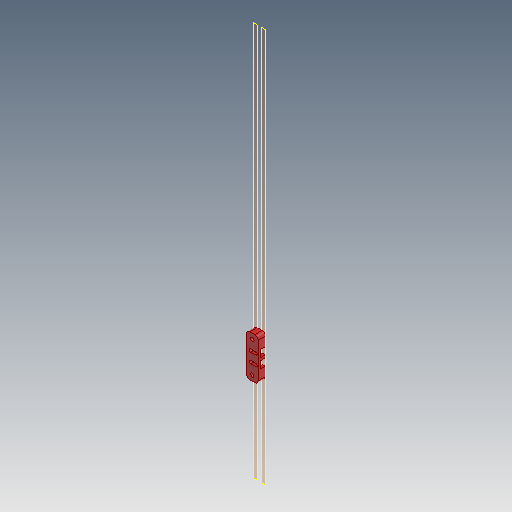
# Autodesk Inventor part: Limit swtich mount bottom
Saved by Autodesk Inventor 2020 (Build 240168000, 168)
## iProperties
Created: 2019-11-21
Part Number: Limit swtich mount bottom
Material: Generic
Document SubType Name: Modeling
Designer: ball
Density: 1 g/cm^3
Appearance: Default
Author: ball
Autodesk Inventor part; units mm, degrees
ref_plane "YZ Plane" through (0, 0, 0) normal (1, 0, 0) x (0, 1, 0)
ref_plane "XZ Plane" through (0, 0, 0) normal (0, 1, 0) x (-1, 0, 0)
ref_plane "Work Plane1" through (0, 0, 0) normal (0, 0, 1) x (1, 0, 0)
ref_plane "Work Plane2" through (0, 0, 0) normal (0, 0, 1) x (1, 0, 0)
sketch "Sketch2" plane through (0, 0, 0) normal (0, 0, 1) x (1, 0, 0)
  line L0 (1.9142, -654.4) -> (1.9142, -1000) construction
  line L1 (13.0858, -1000) -> (13.0858, -654.4) construction
  line L2 (10.8204, -900) -> (1.905, -900) construction
  line L3 (1.1684, -919.8882) -> (10.8204, -919.8882) construction
  circle A0 centre (8.3884, -914.7066) radius 1.1938 construction
  circle A1 centre (8.3884, -905.1816) radius 1.1938 construction
  line L4 (1.9142, -930.0482) -> (13.0858, -930.0482)
  line L5 (13.0858, -930.0482) -> (13.0858, -889.84)
  line L6 (13.0858, -889.84) -> (1.9142, -889.84)
  line L7 (1.9142, -889.84) -> (1.9142, -930.0482)
  circle A2 centre (7.5, -924.8932) radius 1.7
  circle A3 centre (7.5, -894.995) radius 1.7
  circle A4 centre (5.8484, -914.7066) radius 1.4097 construction
  circle A5 centre (5.8484, -914.7066) radius 3.4925 construction
  circle A6 centre (10.9284, -914.7066) radius 1.4097 construction
  circle A7 centre (10.9284, -914.7066) radius 3.4925 construction
  line L8 (5.8484, -914.7066) -> (10.9284, -914.7066) construction
  line L9 (5.8484, -916.1163) -> (10.9284, -916.1163)
  line L10 (10.9284, -913.2969) -> (5.8484, -913.2969)
  arc A8 (5.8484, -913.2969) -> (5.8484, -916.1163) centre (5.8484, -914.7066) ccw
  arc A9 (10.9284, -916.1163) -> (10.9284, -913.2969) centre (10.9284, -914.7066) ccw
  circle A10 centre (10.9284, -905.1816) radius 1.4097 construction
  circle A11 centre (10.9284, -905.1816) radius 3.4925 construction
  line L11 (5.8484, -906.5913) -> (10.9284, -906.5913)
  line L12 (10.9284, -903.7719) -> (5.8484, -903.7719)
  arc A12 (5.8484, -903.7719) -> (5.8484, -906.5913) centre (5.8484, -905.1816) ccw
  arc A13 (10.9284, -906.5913) -> (10.9284, -903.7719) centre (10.9284, -905.1816) ccw
  point P0 (0, 0)
  dimension "d0" = 10.16
  dimension "d1" = 10.16
  dimension "d4" = 3.4
  dimension "d5" = 3.4
  dimension "d6" = 5.155
  dimension "d7" = 5.155
  dimension "d8" = 2.8194
  dimension "d9" = 2.54
  dimension "d10" = 6.985
  dimension "d11" = 2.8194
  dimension "d12" = 6.985
  dimension "d13" = 2.54
  dimension "d14" = 2.8194
  dimension "d15" = 2.8194
  dimension "d16" = 6.985
  dimension "d17" = 2.8194
  constraints: 20 end point, 12 centre point, 8 point on circle, 8 tangent, 4 parallel, 3 coincident, 2 concentric, 2 horizontal, 2 point on line, 1 midpoint, 1 perpendicular
  measures "d0" distance between parallel lines of L4 L3
  measures "d1" distance between parallel lines of L6 L2
  measures "d4" diameter of A2
  measures "d5" diameter of A3
  measures "d6" distance from line of L4 A2.centre
  measures "d7" distance from line of L6 A3.centre
  measures "d8" diameter of A4
  measures "d9" distance of A4.centre A0.centre
  measures "d10" diameter of A5
  measures "d11" diameter of A6
  measures "d12" diameter of A7
  measures "d13" distance of A6.centre A0.centre
  measures "d14" diameter of A9
  measures "d15" diameter of A10
  measures "d16" diameter of A11
  measures "d17" diameter of A13
ref_plane "Work Plane3" through (6.6548, -916.4402, 6.985) normal (0, 0, -1) x (0, 1, 0)
extrude "Extrusion1" add sketch "Sketch2" along normal up to surface (6.985 mm away)
sketch "Sketch3" plane through (0, 0, 0) normal (0, 0, -1) x (-1, 0, 0)
  arc A0 (-5.8484, -906.5913) -> (-5.8484, -903.7719) centre (-5.8484, -905.1816) ccw construction
  arc A1 (-10.9284, -903.7719) -> (-10.9284, -906.5913) centre (-10.9284, -905.1816) ccw construction
  line L0 (-5.8484, -905.1816) -> (-10.9284, -905.1816) construction
  line L1 (-10.9284, -906.5913) -> (-5.8484, -906.5913) construction
  line L2 (-8.3884, -906.5913) -> (-8.3884, -903.7719) construction
  line L3 (-5.8484, -913.2969) -> (-10.9284, -913.2969) construction
  line L4 (-8.3884, -913.2969) -> (-8.3884, -916.1163) construction
  line L5 (-10.9284, -916.1163) -> (-5.8484, -916.1163) construction
  arc A2 (-5.8484, -916.1163) -> (-5.8484, -913.2969) centre (-5.8484, -914.7066) ccw construction
  arc A3 (-10.9284, -913.2969) -> (-10.9284, -916.1163) centre (-10.9284, -914.7066) ccw construction
  line L6 (-5.8484, -914.7066) -> (-10.9284, -914.7066) construction
  line L7 (-13.0858, -930.0482) -> (-13.0858, -889.84) projected
  line L8 (-1.9142, -908.6741) -> (-13.0858, -908.6741)
  line L9 (-13.0858, -908.6741) -> (-13.0858, -901.6891)
  line L10 (-13.0858, -901.6891) -> (-1.9142, -901.6891)
  line L11 (-3.6909, -908.6741) -> (-13.0858, -901.6891) construction
  line L12 (-13.0858, -908.6741) -> (-3.6909, -901.6891) construction
  line L13 (-1.9142, -889.84) -> (-1.9142, -930.0482) construction
  line L14 (-1.9142, -901.6891) -> (-1.9142, -908.6741)
  line L15 (-1.9142, -889.84) -> (-1.9142, -930.0482) projected
  line L16 (-1.9142, -918.1991) -> (-13.0858, -918.1991)
  line L17 (-13.0858, -918.1991) -> (-13.0858, -911.2141)
  line L18 (-13.0858, -911.2141) -> (-1.9142, -911.2141)
  line L19 (-1.9142, -911.2141) -> (-1.9142, -918.1991)
  point P0 (0, 0)
  point P1 (-8.3884, -905.1816)
  dimension "d20" = 6.985
  dimension "d21" = 6.985
  constraints: 28 end point, 6 midpoint, 5 point on line, 4 horizontal, 2 parallel, 2 perpendicular, 1 collinear, 1 vertical
  measures "d20" distance of L8.end L9.end
  measures "d21" distance of L17.start L17.end
extrude "Nut Well" cut sketch "Sketch3" against normal blind 4.572 contours L7 L18 L15 L16 | L7 L10 L14 L8
fillet "Fillet1" radius 3.175 4 edges at (13.0858, -889.84, 3.4925) (13.0858, -930.0482, 3.4925) (1.9142, -930.0482, 3.4925) (1.9142, -889.84, 3.4925)
equation "\"d1\" = d0"
equation "\"d7\" = d6"
body "Solid1"
